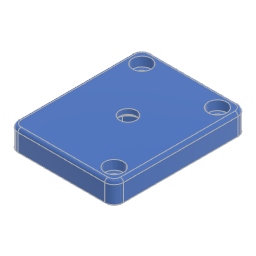
[a]_z_drive_baseplate_a_x2 (Autodesk Fusion 360 design; units mm, degrees)
Autodesk Fusion 360 part; units mm, degrees
sketch "Sketch1" plane through (0, 0, 0) normal (0, 0, 1) x (1, 0, 0) in component "[a]_z_drive_baseplate_a_x2"
  line L0 (16.95, -21.4) -> (-16.95, -21.4)
  line L1 (-16.95, -21.4) -> (-16.95, 21.4)
  line L2 (-16.95, 21.4) -> (16.95, 21.4)
  line L3 (16.95, 21.4) -> (16.95, -21.4)
  line L4 (16.95, -21.4) -> (-16.95, 21.4) construction
  line L5 (-16.95, -21.4) -> (16.95, 21.4) construction
  circle A0 centre (0, 0) radius 2.7
  circle A1 centre (-12.15, 16.6) radius 3
  circle A2 centre (-12.15, 16.6) radius 1.7
  line L6 (4.2, 2.4249) -> (0, 4.8497)
  line L7 (0, 4.8497) -> (-4.2, 2.4249)
  line L8 (-4.2, 2.4249) -> (-4.2, -2.4249)
  line L9 (-4.2, -2.4249) -> (0, -4.8497)
  line L10 (0, -4.8497) -> (4.2, -2.4249)
  line L11 (4.2, -2.4249) -> (4.2, 2.4249)
  line L12 (0, -25) -> (0, 28) construction
  line L13 (-30, 0) -> (30, 0) construction
  circle A3 centre (12.15, 16.6) radius 3
  circle A4 centre (12.15, 16.6) radius 1.7
  circle A5 centre (12.15, -16.6) radius 3
  circle A6 centre (12.15, -16.6) radius 1.7
  circle A7 centre (0, 0) radius 4.1
  dimension "d1" = 33.9
  dimension "d2" = 42.8
  dimension "d3" = 5.4
  dimension "d4" = 6
  dimension "d5" = 4.8
  dimension "d6" = 4.8
  dimension "d7" = 3.4
  dimension "d8" = 4.2
  dimension "d18" = 8.2
  constraint horizontal L0
  constraint perpendicular L0 L1
  constraint parallel L0 L2
  constraint parallel L1 L3
  constraint coincident L4 A0.centre
  constraint coincident L5 A0.centre
  constraint coincident A0.centre A7.centre
  constraint concentric A1 A2
  constraint perpendicular L0 L12
  constraint perpendicular L3 L13
  constraint symmetric A1 L12 A3
  constraint symmetric A2 L12 A4
  constraint symmetric L13 A3 A5
  constraint symmetric L13 A4 A6
  measures "d1" distance of L1.end L2.end
  measures "d2" distance of L0.end L1.end
  measures "d3" diameter of A0
  measures "d4" diameter of A1
  measures "d5" distance of L2 A1.centre
  measures "d6" distance of L1 A1.centre
  measures "d7" diameter of A2
  measures "d8" distance of A0.centre L11
  measures "d18" diameter of A7
extrude "Extrude1" add sketch "Sketch1" along normal mid plane 7 contours L0 L1 L2 L3 | A0 | A1 | A2 | L6 L7 L8 L9 L10 L11 | A3 | A4 | A5 | A6 | A7 in component "[a]_z_drive_baseplate_a_x2"
fillet "Fillet1" radius 3 4 edges at (16.95, -21.4, 0) (-16.95, -21.4, 0) (-16.95, 21.4, 0) (16.95, 21.4, 0) in component "[a]_z_drive_baseplate_a_x2"
extrude "Extrude2" cut sketch "Sketch1" along normal through all and the other way through all contours A0 | A2 | A4 | A6 in component "[a]_z_drive_baseplate_a_x2"
extrude "Extrude3" cut sketch "Sketch1" along normal through all from surface at 0.5 contours A1 | A2 | A3 | A4 | A5 | A6 in component "[a]_z_drive_baseplate_a_x2"
extrude "Extrude4" cut sketch "Sketch1" against normal through all from surface at 0.5 contours A0 | L6 L7 L8 L9 L10 L11 | A7 in component "[a]_z_drive_baseplate_a_x2"
sketch "Sketch2" plane through (0, 0, 0) normal (0, 0, 1) x (1, 0, 0) in component "[a]_z_drive_baseplate_a_x2"
sketch "Sketch3" plane through (0, 0, 0.5) normal (0, 0, -1) x (1, 0, 0) in component "[a]_z_drive_baseplate_a_x2"
  line L0 (4.2, -2.4249) -> (4.2, 2.4249)
  line L1 (4.2, 2.4249) -> (0, 4.8497)
  line L2 (0, 4.8497) -> (-4.2, 2.4249)
  line L3 (-4.2, 2.4249) -> (-4.2, -2.4249)
  line L4 (-4.2, -2.4249) -> (0, -4.8497)
  line L5 (0, -4.8497) -> (4.2, -2.4249)
  circle A0 centre (0, 0) radius 4.1
extrude "Extrude5" cut sketch "Sketch3" against normal through all draft -45 contours A0 in component "[a]_z_drive_baseplate_a_x2"
chamfer "Chamfer1" distance 0.4 angle 45 11 edges at (0, 21.4, -3.5) (16.0713, 20.5213, -3.5) (16.95, 0, -3.5) (16.0713, -20.5213, -3.5) (0, -21.4, -3.5) (-16.0713, -20.5213, -3.5) (-16.95, 0, -3.5) (-16.0713, 20.5213, -3.5) (10.565, 15.9853, -3.5) (10.565, -17.2147, -3.5) (-13.735, 15.9853, -3.5) in component "[a]_z_drive_baseplate_a_x2"
fillet "Fillet2" radius 1 8 edges at (16.0713, 20.5213, 3.5) (0, 21.4, 3.5) (-16.0713, 20.5213, 3.5) (-16.95, 0, 3.5) (-16.0713, -20.5213, 3.5) (0, -21.4, 3.5) (16.0713, -20.5213, 3.5) (16.95, 0, 3.5) in component "[a]_z_drive_baseplate_a_x2"
component "[a]_z_drive_baseplate_a_x2" placed x (1, 0, 0) y (0, 1, 0) z (0, 0, 1) at (0, 0, 0)
